Autodesk Inventor part; units mm, degrees
(part 2 of 2)
  line L320 (-28.6263, 16.0044) -> (-25.6449, 16.0044)
  line L321 (-25.6449, 18.3241) -> (-28.6263, 18.3241)
  line L322 (-29.7503, 19.4482) -> (-24.5209, 19.4482)
  line L323 (-29.5884, 13.8513) -> (-27.9357, 13.8513)
  line L324 (-29.5884, 12.8808) -> (-29.5884, 13.8513)
  line L325 (-29.7503, 14.8804) -> (-29.7503, 19.4482)
  line L326 (-26.6942, 13.8513) -> (-19.7097, 13.8513)
  line L327 (-23.8, 11.9101) -> (-23.8, 12.8808)
  line L328 (-25.8364, 11.9101) -> (-23.8, 11.9101)
  line L329 (-24.7124, 10.786) -> (-24.7124, 8.4664)
  line L330 (-21.731, 8.4664) -> (-21.731, 10.786)
  line L331 (-24.7124, 8.4664) -> (-21.731, 8.4664)
  line L332 (-21.731, 10.786) -> (-24.7124, 10.786)
  line L333 (-26.6942, 14.8804) -> (-26.6942, 13.8513)
  line L334 (-24.5209, 14.8804) -> (-26.6942, 14.8804)
  line L335 (-20.607, 11.9101) -> (-20.607, 7.3423)
  line L336 (-20.607, 7.3423) -> (-25.8364, 7.3423)
  line L337 (-25.8364, 7.3423) -> (-25.8364, 11.9101)
  line L338 (-27.9357, 14.8804) -> (-29.7503, 14.8804)
  line L339 (-37.8438, 41.8417) -> (-37.8438, 39.522)
  line L340 (-41.854, 38.3672) -> (-47.0835, 38.3672)
  line L341 (-45.9594, 39.4913) -> (-42.9781, 39.4913)
  line L342 (-42.9781, 39.4913) -> (-42.9781, 41.8109)
  line L343 (-39.6887, 44.9654) -> (-33.9003, 44.9654)
  line L344 (-43.779, 42.935) -> (-41.854, 42.935)
  line L345 (-42.9781, 41.8109) -> (-45.9594, 41.8109)
  line L346 (-47.8027, 44.9654) -> (-40.8666, 44.9654)
  line L347 (-43.779, 43.9948) -> (-43.779, 42.935)
  line L348 (-44.8621, 42.935) -> (-44.8621, 43.9948)
  line L349 (-47.0835, 42.935) -> (-44.8621, 42.935)
  line L350 (-44.8621, 43.9948) -> (-47.8027, 43.9948)
  line L351 (-45.9594, 41.8109) -> (-45.9594, 39.4913)
  line L352 (-47.0835, 38.3672) -> (-47.0835, 42.935)
  line L353 (-35.553, 43.9948) -> (-35.553, 42.9657)
  line L354 (-40.8666, 44.9654) -> (-40.8666, 45.9361)
  line L355 (-41.854, 42.935) -> (-41.854, 38.3672)
  line L356 (-40.8666, 45.9361) -> (-42.8818, 45.9361)
  line L357 (-47.8027, 43.9948) -> (-47.8027, 44.9654)
  line L358 (-38.9678, 38.398) -> (-38.9678, 42.9657)
  line L359 (-34.8624, 39.522) -> (-34.8624, 41.8417)
  line L360 (-34.8624, 41.8417) -> (-37.8438, 41.8417)
  line L361 (-37.8438, 39.522) -> (-34.8624, 39.522)
  line L362 (-33.7384, 38.398) -> (-38.9678, 38.398)
  line L363 (-33.9003, 43.9948) -> (-35.553, 43.9948)
  line L364 (-33.9003, 44.9654) -> (-33.9003, 43.9948)
  line L365 (-33.7384, 42.9657) -> (-33.7384, 38.398)
  line L366 (-36.7945, 43.9948) -> (-43.779, 43.9948)
  line L367 (-39.6887, 45.9361) -> (-39.6887, 44.9654)
  line L368 (-37.6523, 45.9361) -> (-39.6887, 45.9361)
  line L369 (-38.7764, 47.0601) -> (-38.7764, 49.3798)
  line L370 (-41.7577, 49.3798) -> (-41.7577, 47.0601)
  line L371 (-38.7764, 49.3798) -> (-41.7577, 49.3798)
  line L372 (-41.7577, 47.0601) -> (-38.7764, 47.0601)
  line L373 (-36.7945, 42.9657) -> (-36.7945, 43.9948)
  line L374 (-38.9678, 42.9657) -> (-36.7945, 42.9657)
  line L375 (-42.8818, 45.9361) -> (-42.8818, 50.5038)
  line L376 (-42.8818, 50.5038) -> (-37.6523, 50.5038)
  line L377 (-37.6523, 50.5038) -> (-37.6523, 45.9361)
  line L378 (-35.553, 42.9657) -> (-33.7384, 42.9657)
  line L379 (-40.5846, 75.534) -> (-40.5846, 13.366) construction
  line L380 (-23.2199, 44.9654) -> (-23.2199, 45.9361)
  line L381 (-23.2199, 45.9361) -> (-25.235, 45.9361)
  line L382 (-19.1478, 43.9948) -> (-26.1323, 43.9948)
  line L383 (-24.111, 47.0601) -> (-21.1296, 47.0601)
  line L384 (-20.0056, 45.9361) -> (-22.042, 45.9361)
  line L385 (-24.111, 49.3798) -> (-24.111, 47.0601)
  line L386 (-25.235, 45.9361) -> (-25.235, 50.5038)
  line L387 (-21.1296, 47.0601) -> (-21.1296, 49.3798)
  line L388 (-21.1296, 49.3798) -> (-24.111, 49.3798)
  line L389 (-25.235, 50.5038) -> (-20.0056, 50.5038)
  line L390 (-20.0056, 50.5038) -> (-20.0056, 45.9361)
  line L391 (-22.042, 45.9361) -> (-22.042, 44.9654)
  line L392 (-24.2073, 38.3672) -> (-29.4368, 38.3672)
  line L393 (-28.3127, 39.4913) -> (-25.3314, 39.4913)
  line L394 (-25.3314, 39.4913) -> (-25.3314, 41.8109)
  line L395 (-26.1323, 42.935) -> (-24.2073, 42.935)
  line L396 (-25.3314, 41.8109) -> (-28.3127, 41.8109)
  line L397 (-30.156, 44.9654) -> (-23.2199, 44.9654)
  line L398 (-27.2154, 42.935) -> (-27.2154, 43.9948)
  line L399 (-30.156, 43.9948) -> (-30.156, 44.9654)
  line L400 (-27.2154, 43.9948) -> (-30.156, 43.9948)
  line L401 (-29.4368, 42.935) -> (-27.2154, 42.935)
  line L402 (-28.3127, 41.8109) -> (-28.3127, 39.4913)
  line L403 (-29.4368, 38.3672) -> (-29.4368, 42.935)
  line L404 (-26.1323, 43.9948) -> (-26.1323, 42.935)
  line L405 (-20.1971, 41.8417) -> (-20.1971, 39.522)
  line L406 (-22.042, 44.9654) -> (-16.2536, 44.9654)
  line L407 (-17.9063, 43.9948) -> (-17.9063, 42.9657)
  line L408 (-24.2073, 42.935) -> (-24.2073, 38.3672)
  line L409 (-21.3211, 38.398) -> (-21.3211, 42.9657)
  line L410 (-21.3211, 42.9657) -> (-19.1478, 42.9657)
  line L411 (-19.1478, 42.9657) -> (-19.1478, 43.9948)
  line L412 (-16.2536, 44.9654) -> (-16.2536, 43.9948)
  line L413 (-16.2536, 43.9948) -> (-17.9063, 43.9948)
  line L414 (-17.2157, 41.8417) -> (-20.1971, 41.8417)
  line L415 (-17.9063, 42.9657) -> (-16.0917, 42.9657)
  line L416 (-20.1971, 39.522) -> (-17.2157, 39.522)
  line L417 (-16.0917, 38.398) -> (-21.3211, 38.398)
  line L418 (-16.0917, 42.9657) -> (-16.0917, 38.398)
  line L419 (-17.2157, 39.522) -> (-17.2157, 41.8417)
  line L420 (-29.0148, 57.3686) -> (-29.0148, 55.049)
  line L421 (-33.025, 53.8941) -> (-38.2545, 53.8941)
  line L422 (-37.1304, 55.0182) -> (-34.1491, 55.0182)
  line L423 (-34.1491, 55.0182) -> (-34.1491, 57.3379)
  line L424 (-30.8597, 60.4923) -> (-25.0713, 60.4923)
  line L425 (-34.95, 58.4619) -> (-33.025, 58.4619)
  line L426 (-34.1491, 57.3379) -> (-37.1304, 57.3379)
  line L427 (-38.9737, 60.4923) -> (-32.0376, 60.4923)
  line L428 (-34.95, 59.5218) -> (-34.95, 58.4619)
  line L429 (-36.0331, 58.4619) -> (-36.0331, 59.5218)
  line L430 (-38.2545, 58.4619) -> (-36.0331, 58.4619)
  line L431 (-36.0331, 59.5218) -> (-38.9737, 59.5218)
  line L432 (-37.1304, 57.3379) -> (-37.1304, 55.0182)
  line L433 (-38.2545, 53.8941) -> (-38.2545, 58.4619)
  line L434 (-26.724, 59.5218) -> (-26.724, 58.4927)
  line L435 (-32.0376, 60.4923) -> (-32.0376, 61.463)
  line L436 (-33.025, 58.4619) -> (-33.025, 53.8941)
  line L437 (-32.0376, 61.463) -> (-34.0527, 61.463)
  line L438 (-38.9737, 59.5218) -> (-38.9737, 60.4923)
  line L439 (-30.1388, 53.9249) -> (-30.1388, 58.4927)
  line L440 (-26.0334, 55.049) -> (-26.0334, 57.3686)
  line L441 (-26.0334, 57.3686) -> (-29.0148, 57.3686)
  line L442 (-29.0148, 55.049) -> (-26.0334, 55.049)
  line L443 (-24.9094, 53.9249) -> (-30.1388, 53.9249)
  line L444 (-25.0713, 59.5218) -> (-26.724, 59.5218)
  line L445 (-25.0713, 60.4923) -> (-25.0713, 59.5218)
  line L446 (-24.9094, 58.4927) -> (-24.9094, 53.9249)
  line L447 (-27.9655, 59.5218) -> (-34.95, 59.5218)
  line L448 (-30.8597, 61.463) -> (-30.8597, 60.4923)
  line L449 (-28.8233, 61.463) -> (-30.8597, 61.463)
  line L450 (-29.9473, 62.587) -> (-29.9473, 64.9067)
  line L451 (-32.9287, 64.9067) -> (-32.9287, 62.587)
  line L452 (-29.9473, 64.9067) -> (-32.9287, 64.9067)
  line L453 (-32.9287, 62.587) -> (-29.9473, 62.587)
  line L454 (-27.9655, 58.4927) -> (-27.9655, 59.5218)
  line L455 (-30.1388, 58.4927) -> (-27.9655, 58.4927)
  line L456 (-34.0527, 61.463) -> (-34.0527, 66.0308)
  line L457 (-34.0527, 66.0308) -> (-28.8233, 66.0308)
  line L458 (-28.8233, 66.0308) -> (-28.8233, 61.463)
  line L459 (-26.724, 58.4927) -> (-24.9094, 58.4927)
  spline S0 degree 2 poles (-53.7457, 75.0656) (-54.5032, 75.0656) (-55.7465, 75.5185) (-56.1828, 75.9384) knots 0 0 0 1 2 2 2
  spline S1 degree 2 poles (-56.1828, 75.9384) (-56.611, 76.35) (-57.0556, 77.4698) (-57.0556, 78.1038) knots 0 0 0 1 2 2 2
  spline S2 degree 2 poles (-57.0556, 78.1038) (-57.0556, 78.9271) (-56.1746, 80.3103) (-55.3348, 80.722) knots 0 0 0 1 2 2 2
  line L460 (-55.3348, 80.722) -> (-55.3348, 80.7631)
  spline S3 degree 2 poles (-55.3348, 80.7631) (-56.084, 81.1995) (-56.8086, 82.2369) (-56.8086, 83.0109) knots 0 0 0 1 2 2 2
  spline S4 degree 2 poles (-56.8086, 83.0109) (-56.8086, 84.1553) (-55.0796, 85.6867) (-53.7457, 85.6867) knots 0 0 0 1 2 2 2
  spline S5 degree 2 poles (-53.7457, 85.6867) (-52.3625, 85.6867) (-50.6912, 84.2376) (-50.6912, 83.1014) knots 0 0 0 1 2 2 2
  spline S6 degree 2 poles (-50.6912, 83.1014) (-50.6912, 82.4181) (-51.4898, 81.0842) (-52.239, 80.7055) knots 0 0 0 1 2 2 2
  line L461 (-52.239, 80.7055) -> (-52.239, 80.6643)
  spline S7 degree 2 poles (-52.239, 80.6643) (-51.3498, 80.2527) (-50.4359, 79.0671) (-50.4359, 78.1285) knots 0 0 0 1 2 2 2
  spline S8 degree 2 poles (-50.4359, 78.1285) (-50.4359, 76.8276) (-52.3296, 75.0656) (-53.7457, 75.0656) knots 0 0 0 1 2 2 2
  spline S9 degree 2 poles (-51.8356, 77.9967) (-51.8356, 78.6225) (-52.3296, 79.3635) (-53.0294, 79.7422) knots 0 0 0 1 2 2 2
  spline S10 degree 2 poles (-53.0294, 79.7422) (-53.26, 79.8739) (-54.0339, 80.1786) (-54.5197, 80.3762) knots 0 0 0 1 2 2 2
  spline S11 degree 2 poles (-54.5197, 80.3762) (-55.0796, 80.0057) (-55.6806, 78.9024) (-55.6806, 78.2026) knots 0 0 0 1 2 2 2
  spline S12 degree 2 poles (-55.6806, 78.2026) (-55.6806, 77.2804) (-54.5691, 76.0783) (-53.7293, 76.0783) knots 0 0 0 1 2 2 2
  spline S13 degree 2 poles (-53.7293, 76.0783) (-52.873, 76.0783) (-51.8356, 77.1075) (-51.8356, 77.9967) knots 0 0 0 1 2 2 2
  spline S14 degree 2 poles (-52.025, 83.085) (-52.025, 83.7683) (-52.9389, 84.6822) (-53.754, 84.6822) knots 0 0 0 1 2 2 2
  spline S15 degree 2 poles (-53.754, 84.6822) (-54.495, 84.6822) (-55.4418, 83.8671) (-55.4418, 83.1673) knots 0 0 0 1 2 2 2
  spline S16 degree 2 poles (-55.4418, 83.1673) (-55.4418, 82.6651) (-54.9561, 81.9652) (-54.4703, 81.6853) knots 0 0 0 1 2 2 2
  spline S17 degree 2 poles (-54.4703, 81.6853) (-54.2644, 81.57) (-53.3917, 81.1666) (-53.0377, 81.0513) knots 0 0 0 1 2 2 2
  spline S18 degree 2 poles (-53.0377, 81.0513) (-52.4449, 81.5042) (-52.025, 82.4675) (-52.025, 83.085) knots 0 0 0 1 2 2 2
  spline S19 degree 2 poles (-9.7543, 14.004) (-8.9968, 14.004) (-7.7535, 13.5512) (-7.3172, 13.1313) knots 0 0 0 1 2 2 2
  spline S20 degree 2 poles (-7.3172, 13.1313) (-6.889, 12.7196) (-6.4444, 11.5998) (-6.4444, 10.9659) knots 0 0 0 1 2 2 2
  spline S21 degree 2 poles (-6.4444, 10.9659) (-6.4444, 10.1425) (-7.3254, 8.7593) (-8.1652, 8.3477) knots 0 0 0 1 2 2 2
  line L462 (-8.1652, 8.3477) -> (-8.1652, 8.3065)
  spline S22 degree 2 poles (-8.1652, 8.3065) (-7.416, 7.8701) (-6.6914, 6.8327) (-6.6914, 6.0588) knots 0 0 0 1 2 2 2
  spline S23 degree 2 poles (-6.6914, 6.0588) (-6.6914, 4.9143) (-8.4204, 3.3829) (-9.7543, 3.3829) knots 0 0 0 1 2 2 2
  spline S24 degree 2 poles (-9.7543, 3.3829) (-11.1375, 3.3829) (-12.8088, 4.832) (-12.8088, 5.9682) knots 0 0 0 1 2 2 2
  spline S25 degree 2 poles (-12.8088, 5.9682) (-12.8088, 6.6516) (-12.0102, 7.9854) (-11.261, 8.3641) knots 0 0 0 1 2 2 2
  line L463 (-11.261, 8.3641) -> (-11.261, 8.4053)
  spline S26 degree 2 poles (-11.261, 8.4053) (-12.1502, 8.817) (-13.0641, 10.0026) (-13.0641, 10.9412) knots 0 0 0 1 2 2 2
  spline S27 degree 2 poles (-13.0641, 10.9412) (-13.0641, 12.2421) (-11.1704, 14.004) (-9.7543, 14.004) knots 0 0 0 1 2 2 2
  spline S28 degree 2 poles (-11.6644, 11.0729) (-11.6644, 10.4472) (-11.1704, 9.7062) (-10.4706, 9.3274) knots 0 0 0 1 2 2 2
  spline S29 degree 2 poles (-10.4706, 9.3274) (-10.24, 9.1957) (-9.4661, 8.8911) (-8.9803, 8.6935) knots 0 0 0 1 2 2 2
  spline S30 degree 2 poles (-8.9803, 8.6935) (-8.4204, 9.064) (-7.8194, 10.1672) (-7.8194, 10.8671) knots 0 0 0 1 2 2 2
  spline S31 degree 2 poles (-7.8194, 10.8671) (-7.8194, 11.7892) (-8.9309, 12.9913) (-9.7707, 12.9913) knots 0 0 0 1 2 2 2
  spline S32 degree 2 poles (-9.7707, 12.9913) (-10.627, 12.9913) (-11.6644, 11.9621) (-11.6644, 11.0729) knots 0 0 0 1 2 2 2
  spline S33 degree 2 poles (-11.475, 5.9847) (-11.475, 5.3013) (-10.5611, 4.3874) (-9.746, 4.3874) knots 0 0 0 1 2 2 2
  spline S34 degree 2 poles (-9.746, 4.3874) (-9.005, 4.3874) (-8.0582, 5.2025) (-8.0582, 5.9023) knots 0 0 0 1 2 2 2
  spline S35 degree 2 poles (-8.0582, 5.9023) (-8.0582, 6.4046) (-8.5439, 7.1044) (-9.0297, 7.3844) knots 0 0 0 1 2 2 2
  spline S36 degree 2 poles (-9.0297, 7.3844) (-9.2356, 7.4996) (-10.1083, 7.9031) (-10.4623, 8.0183) knots 0 0 0 1 2 2 2
  spline S37 degree 2 poles (-10.4623, 8.0183) (-11.0551, 7.5655) (-11.475, 6.6022) (-11.475, 5.9847) knots 0 0 0 1 2 2 2
  spline S38 degree 2 poles (-9.7543, 14.004) (-8.9968, 14.004) (-7.7535, 13.5512) (-7.3172, 13.1313) knots 0 0 0 1 2 2 2
  spline S39 degree 2 poles (-7.3172, 13.1313) (-6.889, 12.7196) (-6.4444, 11.5998) (-6.4444, 10.9659) knots 0 0 0 1 2 2 2
  spline S40 degree 2 poles (-6.4444, 10.9659) (-6.4444, 10.1425) (-7.3254, 8.7593) (-8.1652, 8.3477) knots 0 0 0 1 2 2 2
  line L464 (-8.1652, 8.3477) -> (-8.1652, 8.3065)
  spline S41 degree 2 poles (-8.1652, 8.3065) (-7.416, 7.8701) (-6.6914, 6.8327) (-6.6914, 6.0588) knots 0 0 0 1 2 2 2
  spline S42 degree 2 poles (-6.6914, 6.0588) (-6.6914, 4.9143) (-8.4204, 3.3829) (-9.7543, 3.3829) knots 0 0 0 1 2 2 2
  spline S43 degree 2 poles (-9.7543, 3.3829) (-11.1375, 3.3829) (-12.8088, 4.832) (-12.8088, 5.9682) knots 0 0 0 1 2 2 2
  spline S44 degree 2 poles (-12.8088, 5.9682) (-12.8088, 6.6516) (-12.0102, 7.9854) (-11.261, 8.3641) knots 0 0 0 1 2 2 2
  line L465 (-11.261, 8.3641) -> (-11.261, 8.4053)
  spline S45 degree 2 poles (-11.261, 8.4053) (-12.1502, 8.817) (-13.0641, 10.0026) (-13.0641, 10.9412) knots 0 0 0 1 2 2 2
  spline S46 degree 2 poles (-13.0641, 10.9412) (-13.0641, 12.2421) (-11.1704, 14.004) (-9.7543, 14.004) knots 0 0 0 1 2 2 2
  spline S47 degree 2 poles (-11.6644, 11.0729) (-11.6644, 10.4472) (-11.1704, 9.7062) (-10.4706, 9.3274) knots 0 0 0 1 2 2 2
  spline S48 degree 2 poles (-10.4706, 9.3274) (-10.24, 9.1957) (-9.4661, 8.8911) (-8.9803, 8.6935) knots 0 0 0 1 2 2 2
  spline S49 degree 2 poles (-8.9803, 8.6935) (-8.4204, 9.064) (-7.8194, 10.1672) (-7.8194, 10.8671) knots 0 0 0 1 2 2 2
  spline S50 degree 2 poles (-7.8194, 10.8671) (-7.8194, 11.7892) (-8.9309, 12.9913) (-9.7707, 12.9913) knots 0 0 0 1 2 2 2
  spline S51 degree 2 poles (-9.7707, 12.9913) (-10.627, 12.9913) (-11.6644, 11.9621) (-11.6644, 11.0729) knots 0 0 0 1 2 2 2
  spline S52 degree 2 poles (-11.475, 5.9847) (-11.475, 5.3013) (-10.5611, 4.3874) (-9.746, 4.3874) knots 0 0 0 1 2 2 2
  spline S53 degree 2 poles (-9.746, 4.3874) (-9.005, 4.3874) (-8.0582, 5.2025) (-8.0582, 5.9023) knots 0 0 0 1 2 2 2
  spline S54 degree 2 poles (-8.0582, 5.9023) (-8.0582, 6.4046) (-8.5439, 7.1044) (-9.0297, 7.3844) knots 0 0 0 1 2 2 2
  spline S55 degree 2 poles (-9.0297, 7.3844) (-9.2356, 7.4996) (-10.1083, 7.9031) (-10.4623, 8.0183) knots 0 0 0 1 2 2 2
  spline S56 degree 2 poles (-10.4623, 8.0183) (-11.0551, 7.5655) (-11.475, 6.6022) (-11.475, 5.9847) knots 0 0 0 1 2 2 2
  spline S57 degree 2 poles (-53.7457, 75.0656) (-54.5032, 75.0656) (-55.7465, 75.5185) (-56.1828, 75.9384) knots 0 0 0 1 2 2 2
  spline S58 degree 2 poles (-56.1828, 75.9384) (-56.611, 76.35) (-57.0556, 77.4698) (-57.0556, 78.1038) knots 0 0 0 1 2 2 2
  spline S59 degree 2 poles (-57.0556, 78.1038) (-57.0556, 78.9271) (-56.1746, 80.3103) (-55.3348, 80.722) knots 0 0 0 1 2 2 2
  line L466 (-55.3348, 80.722) -> (-55.3348, 80.7631)
  spline S60 degree 2 poles (-55.3348, 80.7631) (-56.084, 81.1995) (-56.8086, 82.2369) (-56.8086, 83.0109) knots 0 0 0 1 2 2 2
  spline S61 degree 2 poles (-56.8086, 83.0109) (-56.8086, 84.1553) (-55.0796, 85.6867) (-53.7457, 85.6867) knots 0 0 0 1 2 2 2
  spline S62 degree 2 poles (-53.7457, 85.6867) (-52.3625, 85.6867) (-50.6912, 84.2376) (-50.6912, 83.1014) knots 0 0 0 1 2 2 2
  spline S63 degree 2 poles (-50.6912, 83.1014) (-50.6912, 82.4181) (-51.4898, 81.0842) (-52.239, 80.7055) knots 0 0 0 1 2 2 2
  line L467 (-52.239, 80.7055) -> (-52.239, 80.6643)
  spline S64 degree 2 poles (-52.239, 80.6643) (-51.3498, 80.2527) (-50.4359, 79.0671) (-50.4359, 78.1285) knots 0 0 0 1 2 2 2
  spline S65 degree 2 poles (-50.4359, 78.1285) (-50.4359, 76.8276) (-52.3296, 75.0656) (-53.7457, 75.0656) knots 0 0 0 1 2 2 2
  spline S66 degree 2 poles (-51.8356, 77.9967) (-51.8356, 78.6225) (-52.3296, 79.3635) (-53.0294, 79.7422) knots 0 0 0 1 2 2 2
  spline S67 degree 2 poles (-53.0294, 79.7422) (-53.26, 79.8739) (-54.0339, 80.1786) (-54.5197, 80.3762) knots 0 0 0 1 2 2 2
  spline S68 degree 2 poles (-54.5197, 80.3762) (-55.0796, 80.0057) (-55.6806, 78.9024) (-55.6806, 78.2026) knots 0 0 0 1 2 2 2
  spline S69 degree 2 poles (-55.6806, 78.2026) (-55.6806, 77.2804) (-54.5691, 76.0783) (-53.7293, 76.0783) knots 0 0 0 1 2 2 2
  spline S70 degree 2 poles (-53.7293, 76.0783) (-52.873, 76.0783) (-51.8356, 77.1075) (-51.8356, 77.9967) knots 0 0 0 1 2 2 2
  spline S71 degree 2 poles (-52.025, 83.085) (-52.025, 83.7683) (-52.9389, 84.6822) (-53.754, 84.6822) knots 0 0 0 1 2 2 2
  spline S72 degree 2 poles (-53.754, 84.6822) (-54.495, 84.6822) (-55.4418, 83.8671) (-55.4418, 83.1673) knots 0 0 0 1 2 2 2
  spline S73 degree 2 poles (-55.4418, 83.1673) (-55.4418, 82.6651) (-54.9561, 81.9652) (-54.4703, 81.6853) knots 0 0 0 1 2 2 2
  spline S74 degree 2 poles (-54.4703, 81.6853) (-54.2644, 81.57) (-53.3917, 81.1666) (-53.0377, 81.0513) knots 0 0 0 1 2 2 2
  spline S75 degree 2 poles (-53.0377, 81.0513) (-52.4449, 81.5042) (-52.025, 82.4675) (-52.025, 83.085) knots 0 0 0 1 2 2 2
  point P0 (-53.7479, 68.8958)
  point P1 (-9.7521, 20.0042)
  point P2 (-41.8348, 101.4209)
  point P3 (-53.7479, 68.8958)
  point P4 (-9.7521, 20.0042)
  point P5 (-1, 6.9835)
  point P6 (-22.9154, 75.534)
  point P7 (-31.7444, 28.893)
  point P8 (-31.7444, 28.893)
  point P9 (-22.9154, 75.534)
  point P10 (-22.9154, 75.534)
  point P11 (-22.9154, 13.366)
  point P12 (-22.9154, 13.366)
  point P13 (-22.9154, 13.366)
  point P14 (-40.5734, 44.4801)
  point P15 (-40.5734, 44.4801)
  point P16 (-22.9266, 44.4801)
  point P17 (-22.9266, 44.4801)
  point P18 (-22.9266, 44.4801)
  point P19 (-31.7444, 60.007)
  point P20 (-31.7444, 60.007)
  point P21 (-31.7444, 60.007)
  point P22 (-31.7444, 28.893)
  dimension "d155" = 8.4153
  dimension "d157" = 0.508
  dimension "d158" = 4.5466
  dimension "d159" = 0.508
  dimension "d160" = 4.5466
  constraints: 894 end point, 50 parallel, 20 perpendicular, 14 horizontal, 5 midpoint, 3 symmetric about line, 1 vertical, 14 other
  measures "d155" distance of L174.end L172.start
  measures "d157" distance between parallel lines of L7 L173
  measures "d158" distance from line of point (-1, 6.983) L172
  measures "d159" distance between parallel lines of L6 L168
  measures "d160" distance between parallel lines of L4 L171
extrude "Extrusion20" add sketch "Sketch17" along normal blind 0.4 contours L48 L49 L73 L71 L76 L69 L86 L79 L85 L67 L62 L68 L84 L80 L87 L77 L82 L60 L55 L61 L81 L78 L83 L70 L75 L72 L74 L50 | L88 L89 L113 L111 L116 L109 L126 L119 L125 L107 L102 L108 L124 L120 L127 L117 L122 L100 L95 L101 L121 L118 L123 L110 L115 L112 L114 L90 | L128 L129 L153 L151 L156 L149 L166 L159 L165 L147 L142 L148 L164 L160 L167 L157 L162 L140 L135 L141 L161 L158 L163 L150 L155 L152 L154 L130 | L179 L185 L186 L189 L190 L191 L194 L192 L193 L209 L207 L208 L217 L216 L197 L198 L199 L195 L206 L205 L204 L201 L215 L214 L218 L188 L183 L184 | L219 L225 L226 L229 L230 L231 L234 L232 L233 L249 L247 L248 L257 L256 L237 L238 L239 L235 L246 L245 L244 L241 L255 L254 L258 L228 L223 L224 | L260 L272 L269 L268 L270 L277 L266 L274 L276 L295 L296 L297 L288 L287 L263 L284 L283 L273 L298 L285 L282 L278 L294 L293 L286 L267 L264 L275 | L300 L312 L309 L308 L310 L317 L306 L314 L316 L335 L336 L337 L328 L327 L303 L324 L323 L313 L338 L325 L322 L318 L334 L333 L326 L307 L304 L315 | L340 L352 L349 L348 L350 L357 L346 L354 L356 L375 L376 L377 L368 L367 L343 L364 L363 L353 L378 L365 L362 L358 L374 L373 L366 L347 L344 L355 | L380 L381 L386 L389 L390 L384 L391 L406 L412 L413 L407 L415 L418 L417 L409 L410 L411 L382 L404 L395 L408 L392 L403 L401 L398 L400 L399 L397 | L421 L433 L430 L429 L431 L438 L427 L435 L437 L456 L457 L458 L449 L448 L424 L445 L444 L434 L459 L446 L443 L439 L455 L454 L447 L428 L425 L436 | S0 S1 S2 L460 S3 S4 S5 S6 L461 S7 S8 | S19 S20 S21 L462 S22 S23 S24 S25 L463 S26 S27 bodies 2
sketch "Sketch18" plane through (0, 0, -0.2) normal (0, 0, -1) x (-1, 0, 0)
  line L0 (0, 0) -> (-63.5, 0)
  line L1 (-63.5, 0) -> (-63.5, 88.9)
  line L2 (-63.5, 88.9) -> (0, 88.9)
  line L3 (0, 88.9) -> (0, 0)
  constraints: 8 end point, 2 parallel, 1 horizontal, 1 perpendicular
extrude "Extrusion21" add sketch "Sketch18" along normal blind 0.4 bodies 3
fillet "Fillet2" radius 3.175 8 edges at (63.5, 0, 0.2) (63.5, 88.9, 0.2) (0, 0, 0.2) (0, 88.9, 0.2) (63.5, 0, -0.3) (63.5, 88.9, -0.3) (0, 0, -0.3) (0, 88.9, -0.3)
extrude "Extrusion22" cut sketch "Sketch17" along normal blind 0.4 contours L48 L49 L73 L71 L76 L69 L86 L79 L85 L67 L62 L68 L84 L80 L87 L77 L82 L60 L55 L61 L81 L78 L83 L70 L75 L72 L74 L50 | L88 L89 L113 L111 L116 L109 L126 L119 L125 L107 L102 L108 L124 L120 L127 L117 L122 L100 L95 L101 L121 L118 L123 L110 L115 L112 L114 L90 | L128 L129 L153 L151 L156 L149 L166 L159 L165 L147 L142 L148 L164 L160 L167 L157 L162 L140 L135 L141 L161 L158 L163 L150 L155 L152 L154 L130 | L179 L185 L186 L189 L190 L191 L194 L192 L193 L209 L207 L208 L217 L216 L197 L198 L199 L195 L206 L205 L204 L201 L215 L214 L218 L188 L183 L184 | L219 L225 L226 L229 L230 L231 L234 L232 L233 L249 L247 L248 L257 L256 L237 L238 L239 L235 L246 L245 L244 L241 L255 L254 L258 L228 L223 L224 | L260 L272 L269 L268 L270 L277 L266 L274 L276 L295 L296 L297 L288 L287 L263 L284 L283 L273 L298 L285 L282 L278 L294 L293 L286 L267 L264 L275 | L300 L312 L309 L308 L310 L317 L306 L314 L316 L335 L336 L337 L328 L327 L303 L324 L323 L313 L338 L325 L322 L318 L334 L333 L326 L307 L304 L315 | L340 L352 L349 L348 L350 L357 L346 L354 L356 L375 L376 L377 L368 L367 L343 L364 L363 L353 L378 L365 L362 L358 L374 L373 L366 L347 L344 L355 | L380 L381 L386 L389 L390 L384 L391 L406 L412 L413 L407 L415 L418 L417 L409 L410 L411 L382 L404 L395 L408 L392 L403 L401 L398 L400 L399 L397 | L421 L433 L430 L429 L431 L438 L427 L435 L437 L456 L457 L458 L449 L448 L424 L445 L444 L434 L459 L446 L443 L439 L455 L454 L447 L428 L425 L436 | S0 S1 S2 L460 S3 S4 S5 S6 L461 S7 S8 | S19 S20 S21 L462 S22 S23 S24 S25 L463 S26 S27 bodies 3
